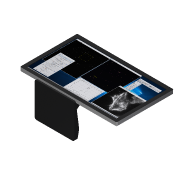
# Autodesk Inventor part: Generic 24pol monitor
Saved by Autodesk Inventor 2019.4 (Build 234330000, 330)
## iProperties
Created: 2017-09-26
Part Number: Generic 24pol monitor
Material: Generic
Document SubType Name: Modeling
Designer: Marcelo
Density: 1 g/cm^3
Appearance: Black Cast(1)
Author: Marcelo
Autodesk Inventor part; units mm, degrees
ref_plane "YZ Plane" through (0, 0, 0) normal (1, 0, 0) x (0, 1, 0)
ref_plane "XZ Plane" through (0, 0, 0) normal (0, 1, 0) x (-1, 0, 0)
ref_plane "XY Plane" through (0, 0, 0) normal (0, 0, 1) x (1, 0, 0)
sketch "Sketch1" plane through (0, 0, 0) normal (1, 0, 0) x (0, 1, 0)
  line L0 (10, 200) -> (30, 50)
  line L1 (30, 50) -> (20, 0)
  line L2 (20, 0) -> (0, 0)
  line L3 (10, 200) -> (0, 200)
  line L4 (0, 200) -> (0, 0)
  dimension "d0" = 10
  dimension "d1" = 20
  dimension "d2" = 150
  dimension "d3" = 200
  dimension "d4" = 30
  constraints: 10 end point, 2 horizontal, 1 coincident, 1 perpendicular
  measures "d0" distance of L0.start L3.end
  measures "d1" distance of L1.end L2.end
  measures "d2" distance from line of L0.end L3
  measures "d3" distance between parallel lines of L2 L3
  measures "d4" distance from line of L4 L0.end
extrude "Extrusion1" add sketch "Sketch1" along normal mid plane 230
sketch "Sketch2" plane through (0, 0, 0) normal (1, 0, 0) x (0, 1, 0)
  line L0 (30, 50) -> (20, 0)
  line L1 (10, 200) -> (30, 50)
  line L2 (30, 50) -> (113.422751, 120)
  line L3 (30, 50) -> (20.588042, 2.940211)
  line L4 (10, 200) -> (0, 200)
  line L5 (160.094466, 120) -> (20.588042, 2.940211)
  line L6 (30, 50) -> (20.588042, 2.940211)
  line L7 (20, 0) -> (30, 50)
  line L8 (0, 0) -> (0, 200)
  line L9 (113.422751, 120) -> (160.094466, 120)
  dimension "d27" = 30
  dimension "d29" = 50
  dimension "d30" = 80
  constraints: 10 end point, 1 collinear, 1 horizontal, 1 parallel, 1 point on line
  measures "d27" distance between parallel lines of L5 L2
  measures "d29" angle of L8 L2
  measures "d30" distance between parallel lines of L9 L4
extrude "Extrusion2" add sketch "Sketch2" along normal mid plane 60
sketch "Sketch7" plane through (0, 0, 0) normal (1, 0, 0) x (0, 1, 0)
  line L0 (80, 140) -> (412, 140)
  line L1 (412, 140) -> (412, 120)
  line L2 (412, 120) -> (80, 120)
  line L3 (80, 140) -> (80, 120)
  line L4 (113.422751, 120) -> (160.094466, 120)
  line L5 (0, 0) -> (0, 200)
  dimension "d31" = 80
  dimension "d32" = 20
  dimension "d33" = 332
  constraints: 8 end point, 3 perpendicular, 1 collinear, 1 horizontal
  measures "d31" distance between parallel lines of L5 L3
  measures "d32" distance between parallel lines of L2 L0
  measures "d33" distance between parallel lines of L3 L1
extrude "Extrusion5" add sketch "Sketch7" along normal mid plane 560
sketch "Sketch9" plane through (280, 412, 120) normal (0, 0, -1) x (-1, 0, 0)
  line L0 (0, 0) -> (560, 0)
  line L1 (0, -332) -> (0, 0)
  line L2 (0, -332) -> (560, -332)
  line L3 (560, 0) -> (560, -332)
  line L4 (310, -298.577249) -> (310, -251.905534)
  line L5 (310, -298.577249) -> (250, -298.577249)
  line L6 (250, -251.905534) -> (250, -298.577249)
  line L7 (310, -251.905534) -> (250, -251.905534)
  point P0 (280, -412)
sketch "Sketch9 outline for Extrusion6" plane through (280, 412, 120) normal (0, 0, -1) x (-1, 0, 0)
  line L0 (560, -332) -> (560, 0)
  line L1 (0, -332) -> (560, -332)
  line L2 (0, 0) -> (0, -332)
  line L3 (560, 0) -> (0, 0)
extrude "Extrusion6" add sketch "Sketch9 outline for Extrusion6" along normal blind 30 draft -60
sketch "Sketch10" plane through (-280, 80, 140) normal (0, 0, 1) x (1, 0, 0)
  line L0 (0, 0) -> (560, 0) projected
  line L1 (560, 332) -> (560, 0) projected
  line L2 (560, 332) -> (0, 332) projected
  line L3 (0, 0) -> (0, 332) projected
  line L4 (20, 312) -> (540, 312)
  line L5 (540, 312) -> (540, 20)
  line L6 (540, 20) -> (20, 20)
  line L7 (20, 20) -> (20, 312)
  point P0 (280, -80)
  dimension "d38" = 20
  constraints: 8 end point, 3 other
  measures "d38" distance between parallel lines of L2 L4
extrude "Extrusion7" cut sketch "Sketch10" against normal blind 3 contours L4 L5 L6 L7
fillet "Fillet4" radius 10 4 edges at (115, 5, 200) (-115, 5, 200) (115, 10, 0) (-115, 10, 0)
fillet "Fillet5" radius 5 4 edges at (280, 412, 130) (280, 80, 130) (-280, 80, 130) (-280, 412, 130)
fillet "Fillet6" radius 20 2 edges at (30, 25.294, 26.4701) (-30, 25.294, 26.4701)
fillet "Fillet7" radius 3 10 edges at (112.0711, 10.3905, 197.0711) (115, 20.6667, 120) (-112.0711, 10.3905, 197.0711) (-115, 20.6667, 120) (0, 10, 200) (112.0711, 20.5858, 2.9289) (0, 20, 0) (-112.0711, 20.5858, 2.9289) (-115, 26, 30) (115, 26, 30)
sketch "Sketch19" plane through (-280, 80, 137) normal (0, 0, 1) x (1, 0, 0)
  line L0 (20, 20) -> (20, 312)
  line L1 (540, 312) -> (540, 20)
  line L2 (20, 312) -> (543.001742, 312) construction
  line L3 (543.001742, 312) -> (543.001742, 26.392032) construction
  line L4 (543.001742, 26.392032) -> (20, 26.392032) construction
  line L5 (20, 26.392032) -> (20, 312) construction
  point P0 (280, -80)
  constraints: 2 other
decal "Decal8"
body "Solid1"
